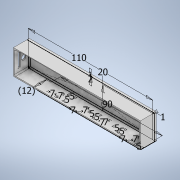
# Autodesk Inventor part: sdm_finger_marker_jig
Saved by Autodesk Inventor 2021 (Build 250183000, 183)
## iProperties
Created: 2021-05-26
Part Number: sdm_finger_marker_jig
Material: Generic
Document SubType Name: Modeling
Designer: Charlie
Density: 1 g/cm^3
Appearance: Default
Author: Charlie
Autodesk Inventor part; units mm, degrees
ref_plane "YZ Plane" through (0, 0, 0) normal (1, 0, 0) x (0, 1, 0)
ref_plane "XZ Plane" through (0, 0, 0) normal (0, 1, 0) x (-1, 0, 0)
ref_plane "XY Plane" through (0, 0, 0) normal (0, 0, 1) x (1, 0, 0)
sketch "Sketch2" plane through (0, 0, 0) normal (0, 0, 1) x (1, 0, 0)
  line L0 (-54, 10) -> (54, 10)
  line L1 (55, 9) -> (55, -9)
  line L2 (54, -10) -> (-54, -10)
  line L3 (-55, -9) -> (-55, 9)
  line L4 (-55, 10) -> (55, -10) construction
  line L5 (55, 10) -> (-55, -10) construction
  line L6 (53, 8) -> (-53, 8)
  line L7 (-53, 8) -> (-53, -8)
  line L8 (-53, -8) -> (53, -8)
  line L9 (53, -8) -> (53, 8)
  line L10 (56, 11) -> (-56, 11)
  line L11 (-56, 11) -> (-56, -11)
  line L12 (-56, -11) -> (56, -11)
  line L13 (56, -11) -> (56, 11)
  arc A0 (55, 9) -> (54, 10) centre (54, 9) ccw
  arc A1 (54, -10) -> (55, -9) centre (54, -9) ccw
  arc A2 (-55, -9) -> (-54, -10) centre (-54, -9) ccw
  arc A3 (-54, 10) -> (-55, 9) centre (-54, 9) ccw
  point P0 (0, 0)
  dimension "d0" = 110
  dimension "d1" = 20
  dimension "d2" = 2
  dimension "d3" = 1
  dimension "d10" = 1
  constraints: 28 end point, 8 point on circle, 8 point on line, 8 tangent, 6 parallel, 4 centre point, 3 equal radius, 3 perpendicular, 2 midpoint, 1 horizontal, 6 other
  measures "d0" distance of L4.end L5.end
  measures "d1" distance of L5.start L4.end
  measures "d2" distance between parallel lines of L0 L6
  measures "d3" distance between parallel lines of L0 L10
  measures "d10" radius of A0
extrude "Extrusion2" add sketch "Sketch2" along normal blind 12 contours L13 L12 L11 L10
sketch "Sketch3" plane through (-56, -11, 0) normal (-1, 0, 0) x (0, 0, 1)
  line L0 (7, 17) -> (9, 17)
  line L1 (9, 17) -> (9, 5)
  line L2 (9, 5) -> (7, 5)
  line L3 (7, 5) -> (7, 17)
  line L4 (0, 22) -> (0, 0) projected
  line L5 (0, 22) -> (12, 22) projected
  circle A0 centre (4, 11) radius 2
  line L6 (12, 22) -> (12, 0) projected
  line L7 (0, 11) -> (2, 11) construction
  dimension "d20" = 4
  dimension "d12" = 2
  dimension "d13" = 12
  dimension "d15" = 5
  dimension "d21" = 3
  dimension "d24" = 4
  dimension "d25" = 2
  dimension "d26" = 3
  constraints: 10 end point, 2 parallel, 1 horizontal, 1 horizontal alignment, 1 perpendicular, 2 other
  measures "d12" distance of L1.end L2.end
  measures "d13" distance of L0.end L1.end
  measures "d15" distance between parallel lines of L5 L0
  measures "d21" distance from line of L3 point (4, 11)
  measures "d24" distance from line of L4 point (4, 11)
  measures "d25" distance of L7.start L7.end
  measures "d26" distance between parallel lines of L6 L1
extrude "Extrusion4" cut sketch "Sketch3" against normal blind 10
extrude "Extrusion5" add sketch "Sketch2" against normal blind 2 contours L0 A0 L1 A1 L2 A2 L3 A3 | L9 L8 L7 L6 | L13 L12 L11 L10
sketch "Sketch4" plane through (-54, 10, 12) normal (0, -1, 0) x (1, 0, 0)
  line L0 (3.4899, -1) -> (43.4899, -1)
  line L1 (43.4899, -1) -> (43.4899, 0)
  line L2 (43.4899, 0) -> (3.4899, 0)
  line L3 (3.4899, 0) -> (3.4899, -1)
  line L4 (0, 0) -> (108, 0) projected
  point P0 (54, -12)
  dimension "d27" = 1
  dimension "d28" = 40
  constraints: 8 end point, 2 parallel, 1 horizontal, 1 perpendicular, 1 point on line
  measures "d27" distance of L2.end L0.start
  measures "d28" distance of L1.end L2.end
extrude "Extrusion6" cut sketch "Sketch4" against normal blind 0.5
sketch "Sketch5" plane through (-56, -11, 12) normal (0, -1, 0) x (1, 0, 0)
  line L0 (111, -12) -> (111, 0) construction
  line L1 (111, -6) -> (1, -6) construction
  line L2 (1, -12) -> (1, 0) construction
  line L3 (38.5, -3.5) -> (38.5, -8.5)
  line L4 (38.5, -8.5) -> (43.5, -8.5)
  line L5 (43.5, -8.5) -> (43.5, -3.5)
  line L6 (43.5, -3.5) -> (38.5, -3.5)
  line L7 (38.5, -3.5) -> (43.5, -8.5) construction
  line L8 (38.5, -8.5) -> (43.5, -3.5) construction
  line L9 (26.5, -9.5) -> (26.5, -2.5)
  line L10 (26.5, -2.5) -> (33.5, -2.5)
  line L11 (33.5, -2.5) -> (33.5, -9.5)
  line L12 (33.5, -9.5) -> (26.5, -9.5)
  line L13 (26.5, -9.5) -> (33.5, -2.5) construction
  line L14 (26.5, -2.5) -> (33.5, -9.5) construction
  line L15 (60.4912, -8.5) -> (65.4912, -8.5)
  line L16 (65.4912, -8.5) -> (65.4912, -3.5)
  line L17 (65.4912, -3.5) -> (60.4912, -3.5)
  line L18 (60.4912, -3.5) -> (65.4912, -8.5) construction
  line L19 (60.4912, -3.5) -> (60.4912, -8.5)
  line L20 (60.4912, -8.5) -> (65.4912, -3.5) construction
  line L21 (55.4912, -9.5) -> (48.4912, -9.5)
  line L22 (48.4912, -9.5) -> (48.4912, -2.5)
  line L23 (55.4912, -2.5) -> (55.4912, -9.5)
  line L24 (48.4912, -9.5) -> (55.4912, -2.5) construction
  line L25 (48.4912, -2.5) -> (55.4912, -9.5) construction
  line L26 (48.4912, -2.5) -> (55.4912, -2.5)
  line L27 (77.5, -9.5) -> (70.5, -9.5)
  line L28 (77.5, -2.5) -> (77.5, -9.5)
  line L29 (70.5, -2.5) -> (77.5, -2.5)
  line L30 (70.5, -2.5) -> (77.5, -9.5) construction
  line L31 (70.5, -9.5) -> (70.5, -2.5)
  line L32 (70.5, -9.5) -> (77.5, -2.5) construction
  line L33 (82.5, -3.5) -> (82.5, -8.5)
  line L34 (87.5, -3.5) -> (82.5, -3.5)
  line L35 (82.5, -3.5) -> (87.5, -8.5) construction
  line L36 (82.5, -8.5) -> (87.5, -3.5) construction
  line L37 (87.5, -8.5) -> (87.5, -3.5)
  line L38 (82.5, -8.5) -> (87.5, -8.5)
  line L39 (99.5, -9.5) -> (92.5, -9.5)
  line L40 (99.5, -2.5) -> (99.5, -9.5)
  line L41 (92.5, -2.5) -> (99.5, -2.5)
  line L42 (92.5, -2.5) -> (99.5, -9.5) construction
  line L43 (92.5, -9.5) -> (92.5, -2.5)
  line L44 (92.5, -9.5) -> (99.5, -2.5) construction
  line L45 (106, -6) -> (30, -6) construction
  line L46 (110, 0) -> (111, 0) projected
  line L47 (110, -12) -> (2, -12) projected
  line L48 (111, 0) -> (21, 0)
  line L49 (21, 0) -> (21, -12)
  line L50 (21, -12) -> (111, -12)
  line L51 (111, -12) -> (111, 0)
  line L52 (112, -14) -> (112, 0) projected
  line L53 (111, 0) -> (112, 0)
  line L54 (112, 0) -> (112, -14)
  line L55 (112, -14) -> (21, -14)
  line L56 (0, -14) -> (112, -14) projected
  line L57 (21, -14) -> (21, -12)
  point P0 (41, -6)
  point P1 (62.9912, -6)
  point P2 (51.9912, -6)
  point P3 (74, -6)
  point P4 (85, -6)
  point P5 (96, -6)
  dimension "d47" = 5
  dimension "d48" = 5
  dimension "d49" = 7
  dimension "d50" = 7
  dimension "d51" = 5
  dimension "d52" = 5
  dimension "d53" = 7
  dimension "d54" = 7
  dimension "d55" = 5
  dimension "d56" = 5
  dimension "d57" = 7
  dimension "d58" = 7
  dimension "d59" = 7
  dimension "d60" = 7
  dimension "d61" = 5
  dimension "d62" = 90
  dimension "d63" = 12
  constraints: 104 end point, 16 midpoint, 3 equal length, 3 point on line, 2 horizontal, 2 perpendicular
  measures "d47" distance of L5.end L5.start
  measures "d48" distance of L5.start L4.start
  measures "d49" distance of L13.end L12.start
  measures "d50" distance of L9.end L13.end
  measures "d51" distance of L16.end L15.end
  measures "d52" distance of L15.end L15.start
  measures "d53" distance of L23.start L21.start
  measures "d54" distance of L22.end L23.start
  measures "d55" distance of L36.end L38.end
  measures "d56" distance of L38.end L33.end
  measures "d57" distance of L28.start L27.start
  measures "d58" distance of L29.start L28.start
  measures "d59" distance of L41.end L40.end
  measures "d60" distance of L41.start L41.end
  measures "d61" distance from line of L0 point (106, -6)
  measures "d62" distance of L50.end L49.end
  measures "d63" distance of L48.end L49.end
body "Solid1"
